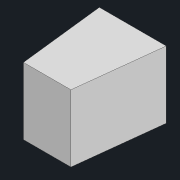
# Autodesk Inventor part: Cap
Saved by Autodesk Inventor 2022.3 (Build 263350000, 350)
## iProperties
Created: 2022-10-27
Part Number: Cap
Material: Generic
Document SubType Name: Modeling
Designer: JARRETT
Density: 1 g/cm^3
Appearance: Default
Author: JARRETT
Autodesk Inventor part; units mm, degrees
ref_plane "YZ Plane" through (0, 0, 0) normal (1, 0, 0) x (0, 1, 0)
ref_plane "XZ Plane" through (0, 0, 0) normal (0, 1, 0) x (-1, 0, 0)
ref_plane "XY Plane" through (0, 0, 0) normal (0, 0, 1) x (1, 0, 0)
sketch "Sketch1" plane through (0, 0, 0) normal (0, 1, 0) x (-1, 0, 0)
  line L0 (9, 16.2464) -> (-9, 16.2464)
  line L1 (-9, 16.2464) -> (-12.7, -16.2464)
  line L2 (-12.7, -16.2464) -> (12.7, -16.2464)
  line L3 (12.7, -16.2464) -> (9, 16.2464)
  line L4 (0, -16.2464) -> (0, 16.2464)
  point P0 (0, 0)
  point P1 (0, 0)
  dimension "d6" = 18
  dimension "d27" = 25.4
  constraints: 10 end point, 4 midpoint, 1 coincident, 1 horizontal, 1 parallel, 1 perpendicular, 1 point on line
  measures "d6" distance of L0.start L0.end
  measures "d27" distance of L1.end L2.end
extrude "Extrusion1" add sketch "Sketch1" along normal blind 25.4
body "Solid2"
